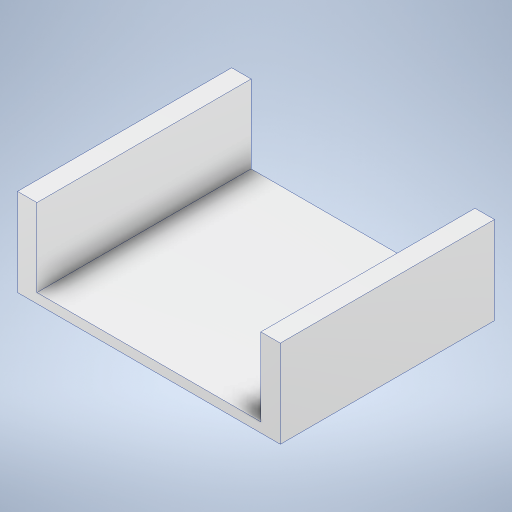
# Autodesk Inventor part: Podkladka
Saved by Autodesk Inventor 2024 (Build 280153000, 153)
## iProperties
Created: 2023-08-16
Part Number: Podkladka
Material: Aluminum 6061
Document SubType Name: Modeling
Designer: Kippi
Density: 2.7 g/cm^3
Appearance: Aluminum - Flat
Mass: 3504.6 g
Surface Area: 2054 cm^2
Volume: 1298 cm^3
Author: Kippi
Autodesk Inventor part; units mm, degrees
ref_plane "YZ Plane" through (0, 0, 0) normal (1, 0, 0) x (0, 1, 0)
ref_plane "XZ Plane" through (0, 0, 0) normal (0, 1, 0) x (-1, 0, 0)
ref_plane "XY Plane" through (0, 0, 0) normal (0, 0, 1) x (1, 0, 0)
sketch "Sketch1" plane through (0, 0, 0) normal (0, 1, 0) x (-1, 0, 0)
  line L0 (86.4286, 125.7143) -> (-143.5714, 125.7143)
  line L1 (-143.5714, 125.7143) -> (-143.5714, -94.2857)
  line L2 (-143.5714, -94.2857) -> (86.4286, -94.2857)
  line L3 (86.4286, -94.2857) -> (86.4286, 125.7143)
  point P0 (0, 0)
  dimension "d0" = 220
  dimension "d1" = 230
  constraints: 8 end point, 2 parallel, 1 horizontal, 1 perpendicular
  measures "d0" distance of L2.end L0.start
  measures "d1" distance of L1.end L2.end
extrude "Extrusion1" add sketch "Sketch1" along normal blind 10
sketch "Sketch5" plane through (-86.4286, 0, 125.7143) normal (0, 0, 1) x (1, 0, 0)
  line L0 (0, 0) -> (0, 10) projected
  line L1 (0, 0) -> (-20, 0)
  line L2 (-20, 0) -> (-20, 90)
  line L3 (-20, 90) -> (0, 90)
  line L4 (0, 90) -> (0, 0)
  line L5 (230, 0) -> (0, 0) projected
  line L6 (230, 0) -> (250, 0)
  line L7 (250, 0) -> (250, 90)
  line L8 (250, 90) -> (230, 90)
  line L9 (230, 90) -> (230, 0)
  point P0 (86.4286, 0)
  dimension "d22" = 90
  dimension "d23" = 20
  dimension "d24" = 20
  constraints: 16 end point, 4 parallel, 2 horizontal, 2 perpendicular, 1 collinear
  measures "d22" distance between parallel lines of L5 L3
  measures "d23" distance of L5.start L6.end
  measures "d24" distance of L0.start L1.end
extrude "Extrusion5" add sketch "Sketch5" against normal up to surface (220 mm away)
body "Solid1"
